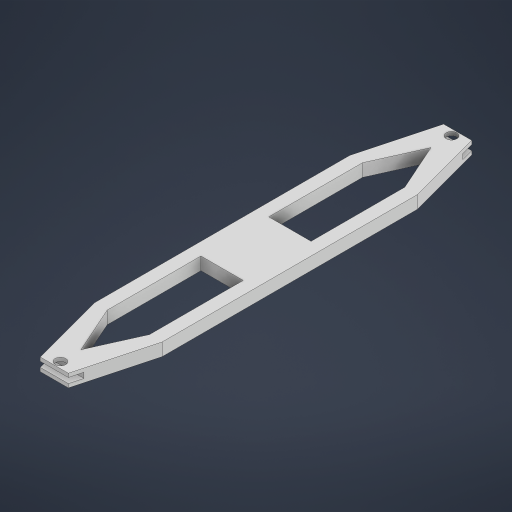
# Autodesk Inventor part: Diff_BarV2
Saved by Autodesk Inventor 2023 (Build 270158000, 158)
## iProperties
Created: 2023-04-06
Part Number: Diff_BarV2
Material: Generic
Document SubType Name: Modeling
Designer: bugme
Density: 1 g/cm^3
Appearance: Default
Author: bugme
Autodesk Inventor part; units mm, degrees
ref_plane "YZ Plane" through (0, 0, 0) normal (1, 0, 0) x (0, 1, 0)
ref_plane "XZ Plane" through (0, 0, 0) normal (0, 1, 0) x (-1, 0, 0)
ref_plane "XY Plane" through (0, 0, 0) normal (0, 0, 1) x (1, 0, 0)
sketch "Sketch1" plane through (0, 0, 0) normal (0, 1, 0) x (-1, 0, 0)
  line L0 (50.8, 0) -> (50.8, -300)
  line L1 (50.8, -300) -> (-50.8, -300)
  line L2 (-50.8, -300) -> (-50.8, 0)
  line L3 (50.8, 0) -> (50.8, 300)
  line L4 (50.8, 300) -> (-50.8, 300)
  line L5 (-50.8, 300) -> (-50.8, 0)
  line L6 (0, -420) -> (0, 420) projected
  line L7 (31.75, 280.95) -> (31.75, 50.8)
  line L8 (31.75, -50.8) -> (31.75, -280.95)
  line L9 (31.75, -280.95) -> (-31.75, -280.95)
  line L10 (-31.75, -280.95) -> (-31.75, -50.8)
  line L11 (-31.75, 50.8) -> (-31.75, 280.95)
  line L12 (-31.75, 280.95) -> (31.75, 280.95)
  line L13 (71.12, 0) -> (-71.12, 0) projected
  line L14 (31.75, 50.8) -> (-31.75, 50.8)
  line L15 (31.75, -50.8) -> (-31.75, -50.8)
  dimension "d15" = 101.6
  dimension "d19" = 600
  dimension "d20" = 19.05
  dimension "d22" = 101.6
  constraints: 28 end point, 4 equal length, 4 perpendicular, 2 symmetric about line, 1 horizontal, 1 vertical, 1 vertical alignment, 1 other
  measures "d15" distance of L3.end L4.end
  measures "d19" distance of L0.end L3.end
  measures "d20" distance between parallel lines of L3 L7
  measures "d22" distance between parallel lines of L15 L14
extrude "Extrusion1" add sketch "Sketch1" along normal blind 19.05 contours L13 L6 L14 L7 L12 L4 L3 | L0 L1 L6 L9 L8 L15 L13 | L13 L5 L4 L6 L12 L11 L14 | L6 L15 L10 L9 L1 L2 L13
sketch "Sketch4" plane through (0, 19.05, 0) normal (0, 1, 0) x (1, 0, 0)
  line L0 (-50.8, 300) -> (-50.8, -300) projected
  line L1 (-50.8, -300) -> (50.8, -300) projected
  line L2 (-50.8, -191.4687) -> (61.5598, -191.4687) construction
  line L3 (-50.8, -191.4687) -> (50.8, -191.4687)
  line L4 (0, 422.6237) -> (0, -422.6237) projected
  line L5 (-50.8, -191.4687) -> (50.8, -191.4687)
  line L6 (50.8, -300) -> (50.8, 300) projected
  line L7 (-50.8, -191.4687) -> (-21.217, -301.8741)
  line L8 (-50.8, -191.4687) -> (63.5, -191.4687) construction
  line L9 (50.8, -191.4687) -> (21.217, -301.8741)
  line L10 (-21.217, -301.8741) -> (21.217, -301.8741)
  line L11 (-21.7191, -300) -> (21.7191, -300)
  line L12 (-73.66, 0) -> (86.36, 0) projected
  line L13 (-50.8, 300) -> (50.8, 300)
  line L14 (-50.8, 191.4687) -> (61.5598, 191.4687) construction
  line L15 (-50.8, 191.4687) -> (50.8, 191.4687)
  line L16 (-50.8, 191.4687) -> (50.8, 191.4687)
  line L17 (-50.8, 191.4687) -> (-21.217, 301.8741)
  line L18 (-50.8, 191.4687) -> (63.5, 191.4687) construction
  line L19 (50.8, 191.4687) -> (21.217, 301.8741)
  line L20 (-21.217, 301.8741) -> (21.217, 301.8741)
  line L21 (-21.7191, 300) -> (21.7191, 300)
  line L22 (-31.75, -280.95) -> (-31.75, -50.8) projected
  line L23 (31.75, -280.95) -> (-31.75, -280.95) projected
  line L24 (31.75, -50.8) -> (31.75, -280.95) projected
  line L25 (-31.75, 50.8) -> (-31.75, 280.95) projected
  line L26 (-31.75, 280.95) -> (31.75, 280.95) projected
  line L27 (31.75, 280.95) -> (31.75, 50.8) projected
  point P0 (0, 0)
  point P1 (-26.8236, 280.95)
  point P2 (-31.75, 262.5643)
  point P3 (31.75, 262.5643)
  point P4 (26.8236, 280.95)
  point P5 (31.75, -262.5643)
  point P6 (26.8236, -280.95)
  point P7 (-26.8236, -280.95)
  point P8 (-31.75, -262.5643)
  dimension "d28" = 114.3
  dimension "d29" = 75
  constraints: 34 end point, 11 point on line, 9 symmetric about line, 3 horizontal, 1 equal length, 1 perpendicular
  measures "d28" distance of L2.start L7.end
  measures "d29" angle of L7 L8
extrude "Extrusion4" cut sketch "Sketch4" against normal blind 25.4 contours L13 L17 L26 L25 L0 | L7 L22 L23 L1 L0 | L13 L6 L19 L27 L26 | L6 L1 L9 L23 L24
sketch "Sketch5" plane through (0, 19.05, 0) normal (0, 1, 0) x (1, 0, 0)
  line L0 (26.8236, -280.95) -> (-26.8236, -280.95) projected
  line L1 (-31.75, -262.5643) -> (-26.8236, -280.95)
  line L2 (-26.8236, -280.95) -> (26.8236, -280.95)
  line L3 (31.75, -50.8) -> (31.75, -262.5643) projected
  line L4 (26.8236, -280.95) -> (31.75, -262.5643)
  line L5 (31.75, -262.5643) -> (-31.75, -262.5643)
  line L6 (21.7191, -300) -> (-21.7191, -300) projected
  line L7 (21.7191, -300) -> (21.0617, -302.4535)
  line L8 (21.0617, -302.4535) -> (-21.0617, -302.4535)
  line L9 (-21.0617, -302.4535) -> (-21.7191, -300)
  line L10 (-71.12, 0) -> (71.12, 0) projected
  line L11 (26.8236, 280.95) -> (-26.8236, 280.95)
  line L12 (-31.75, 262.5643) -> (-26.8236, 280.95)
  line L13 (-26.8236, 280.95) -> (26.8236, 280.95)
  line L14 (26.8236, 280.95) -> (31.75, 262.5643)
  line L15 (31.75, 262.5643) -> (-31.75, 262.5643)
  line L16 (21.7191, 300) -> (-21.7191, 300)
  line L17 (21.7191, 300) -> (21.0617, 302.4535)
  line L18 (21.0617, 302.4535) -> (-21.0617, 302.4535)
  line L19 (-21.0617, 302.4535) -> (-21.7191, 300)
  point P0 (0, 0)
  dimension "d32" = 2.54
  constraints: 32 end point, 8 symmetric about line, 4 point on line, 2 collinear, 1 parallel, 1 perpendicular
  measures "d32" distance of L6.start L7.end
extrude "Extrusion5" add sketch "Sketch5" against normal up to surface (19.05 mm away)
sketch "Sketch6" plane through (0, 19.05, 0) normal (0, 1, 0) x (1, 0, 0)
  line L0 (-50.8, 191.4687) -> (-50.8, -191.4687) projected
  line L1 (-50.8, -191.4687) -> (-31.75, -191.4687)
  line L2 (-31.75, -262.5643) -> (-31.75, -50.8) projected
  line L3 (-31.75, -191.4687) -> (0, -262.5643)
  line L4 (31.75, -262.5643) -> (-31.75, -262.5643) projected
  line L5 (50.8, -191.4687) -> (50.8, 191.4687) projected
  line L6 (50.8, -191.4687) -> (31.75, -191.4687)
  line L7 (31.75, -50.8) -> (31.75, -262.5643) projected
  line L8 (31.75, -191.4687) -> (0, -262.5643)
  line L9 (-71.12, 0) -> (71.12, 0) projected
  line L10 (31.75, -191.4687) -> (31.75, -262.5643)
  line L11 (0, -262.5643) -> (31.75, -262.5643)
  line L12 (0, -262.5643) -> (-31.75, -262.5643)
  line L13 (-31.75, -191.4687) -> (-31.75, -262.5643)
  line L14 (-50.8, 191.4687) -> (-31.75, 191.4687)
  line L15 (-31.75, 191.4687) -> (0, 262.5643)
  line L16 (31.75, 262.5643) -> (-31.75, 262.5643)
  line L17 (50.8, 191.4687) -> (31.75, 191.4687)
  line L18 (31.75, 191.4687) -> (0, 262.5643)
  line L19 (31.75, 191.4687) -> (31.75, 262.5643)
  line L20 (0, 262.5643) -> (31.75, 262.5643)
  line L21 (0, 262.5643) -> (-31.75, 262.5643)
  line L22 (-31.75, 191.4687) -> (-31.75, 262.5643)
  point P0 (0, 0)
  constraints: 34 end point, 5 symmetric about line, 4 collinear, 4 point on line, 1 horizontal, 1 midpoint
extrude "Extrusion6" add sketch "Sketch6" against normal up to surface (19.05 mm away) contours L22 L16 L15 | L16 L19 L18 | L3 L4 L2 | L8 L7 L4
sketch "Sketch7" plane through (50.8, 0, 191.4687) normal (1, 0, 0) x (0, 0, -1)
  line L0 (382.9375, 19.05) -> (493.9222, 19.05) projected
  line L1 (493.9222, 0) -> (382.9375, 0) projected
  line L2 (614.9036, 0) -> (-231.9661, 0) projected
  line L3 (493.9222, 19.05) -> (493.9222, 0) projected
  line L4 (493.9222, 19.05) -> (493.9222, 0)
  line L5 (493.9222, 0) -> (493.9222, 9.525)
  line L6 (493.9222, 13.4938) -> (493.9222, 5.5563)
  line L7 (493.9222, 13.4938) -> (475.5072, 13.4938)
  line L8 (475.5072, 13.4938) -> (475.5072, 5.5563)
  line L9 (475.5072, 5.5563) -> (493.9222, 5.5563)
  line L10 (191.4687, -3.81) -> (191.4687, 22.86) projected
  line L11 (-110.9847, 13.4938) -> (-110.9847, 5.5563)
  line L12 (-110.9847, 13.4938) -> (-92.5697, 13.4938)
  line L13 (-92.5697, 13.4938) -> (-92.5697, 5.5563)
  line L14 (-92.5697, 5.5563) -> (-110.9847, 5.5563)
  point P0 (191.4687, 0)
  point P1 (-110.9847, 9.525)
  dimension "d39" = 7.9375
  dimension "d40" = 18.415
  constraints: 20 end point, 5 symmetric about line, 3 perpendicular, 2 point on line, 1 collinear, 1 midpoint
  measures "d39" distance of L6.start L6.end
  measures "d40" distance of L6.start L7.end
extrude "Extrusion7" cut sketch "Sketch7" against normal through all
sketch "Sketch8" plane through (0, 19.05, 0) normal (0, 1, 0) x (1, 0, 0)
  line L0 (25.996, -284.0385) -> (-25.996, -284.0385) projected
  line L1 (-21.0617, -302.4535) -> (21.0617, -302.4535) projected
  circle A0 centre (0, -293.246) radius 7.9375
  line L2 (-71.12, 0) -> (71.12, 0) projected
  circle A1 centre (0, 293.246) radius 7.9375
  point P0 (0, 0)
  dimension "d43" = 15.875
  constraints: 2 centre point, 1 symmetric about line, 1 other
  measures "d43" diameter of A0
extrude "Extrusion8" cut sketch "Sketch8" against normal up to surface (13.4938 mm away)
body "Solid1"
